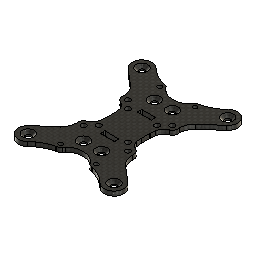
T_v2_Bottom_Plate_7_Inch_3mm (Autodesk Fusion 360 design; units mm, degrees)
Autodesk Fusion 360 part; units mm, degrees
sketch "Bottom Plate v2 3mm" plane through (0, 0, 0) normal (0, 0, 1) x (1, 0, 0)
  line L0 (23.8549, 2.6173) -> (23.8549, 4.2)
  arc A0 (38.0902, -44.8281) -> (37.3115, -43.7825) centre (33.725, -47.2663) ccw
  arc A1 (3.5774, -53.5563) -> (-5.1954, -43.2296) centre (-0.8133, -48.3966) cw
  arc A2 (24.6115, 1.8607) -> (23.8549, 2.6173) centre (24.2332, 2.239) cw
  line L1 (32.7104, -23.5665) -> (24.6115, -23.5665)
  arc A3 (16.0943, -15.706) -> (16.4474, -12.2676) centre (-17.5938, -10.5095) ccw
  arc A4 (40.5915, -46.4096) -> (38.0902, -44.8281) centre (40.7966, -43.3163) cw
  circle A5 centre (34.8621, 15.0393) radius 1.95
  arc A6 (23.8549, 4.2) -> (24.6115, 4.9567) centre (24.2332, 4.5783) cw
  arc A7 (41.2277, -2.9039) -> (40.8746, -6.3422) centre (74.9158, -8.1003) ccw
  line L2 (24.6115, -20.4705) -> (32.7104, -20.4705)
  arc A8 (47.7927, -25.5206) -> (51.1194, -33.5105) centre (59.6599, -25.267) ccw
  arc A9 (20.0105, 25.1727) -> (37.3115, 25.1727) centre (28.661, 33.5756) ccw
  arc A10 (24.6115, -23.5665) -> (23.8549, -22.8099) centre (24.2332, -23.1882) cw
  circle A11 centre (18.661, 0.6951) radius 1.75
  arc A12 (40.8746, -12.2676) -> (41.2277, -15.706) centre (74.9158, -10.5095) ccw
  line L3 (24.6115, 4.9567) -> (32.7104, 4.9567)
  arc A13 (33.467, 2.6173) -> (32.7104, 1.8607) centre (33.0887, 2.239) cw
  arc A14 (40.8746, -6.3422) -> (40.8775, -6.4049) centre (74.188, -4.8447) ccw
  arc A15 (23.8549, -21.2271) -> (24.6115, -20.4705) centre (24.2332, -20.8488) cw
  arc A16 (16.1379, -46.4846) -> (6.6741, -50.9212) centre (21.6796, -70.6178) ccw
  arc A17 (6.2139, -33.5209) -> (9.5318, -25.5307) centre (-2.3021, -25.3006) ccw
  circle A18 centre (38.661, 0.6951) radius 1.75
  arc A19 (-5.2039, 24.6271) -> (3.5715, 34.9515) centre (-0.8144, 29.7877) cw
  arc A20 (37.3115, -43.7825) -> (20.0105, -43.7825) centre (28.661, -52.1854) ccw
  circle A21 centre (22.4599, -33.6491) radius 1.95
  arc A22 (33.467, -22.8099) -> (32.7104, -23.5665) centre (33.0887, -23.1882) cw
  arc A23 (16.4474, -6.3422) -> (16.0943, -2.9039) centre (-17.5938, -8.1003) ccw
  line L4 (33.467, 4.2) -> (33.467, 2.6173)
  circle A24 centre (22.4599, 15.0393) radius 1.95
  line L5 (23.8549, -22.8099) -> (23.8549, -21.2271)
  circle A25 centre (38.661, -19.3049) radius 1.75
  arc A26 (40.8775, -12.2049) -> (40.8746, -12.2676) centre (74.188, -13.7651) ccw
  circle A27 centre (-0.8133, -48.3966) radius 1.95
  arc A28 (11.677, 2.3405) -> (9.5318, 6.9209) centre (13.411, 5.9451) cw
  arc A29 (53.7651, 34.9349) -> (62.5417, 24.6115) centre (58.1639, 29.7821) cw
  circle A30 centre (18.661, -19.3049) radius 1.75
  line L6 (32.7104, 1.8607) -> (24.6115, 1.8607)
  arc A31 (37.3115, 25.1727) -> (38.0902, 26.2183) centre (33.725, 28.6565) ccw
  arc A32 (19.2318, 26.2183) -> (20.0105, 25.1727) centre (23.5969, 28.6565) ccw
  arc A33 (32.7104, 4.9567) -> (33.467, 4.2) centre (33.0887, 4.5783) cw
  arc A34 (16.7304, 27.7997) -> (19.2318, 26.2183) centre (16.5253, 24.7065) cw
  arc A35 (45.6449, -20.9503) -> (47.7927, -25.5206) centre (43.911, -24.5549) cw
  arc A36 (32.7104, -20.4705) -> (33.467, -21.2271) centre (33.0887, -20.8488) cw
  circle A37 centre (43.911, -24.5549) radius 1.75
  circle A38 centre (43.911, 5.9451) radius 1.75
  line L7 (62.5417, 24.6115) -> (51.1194, 14.9007)
  line L8 (53.7651, -53.5447) -> (50.661, -50.9058)
  arc A39 (47.7927, 6.9108) -> (45.6449, 2.3405) centre (43.911, 5.9451) cw
  line L9 (33.467, -21.2271) -> (33.467, -22.8099)
  circle A40 centre (13.411, 5.9451) radius 1.75
  line L10 (-5.1954, -43.2296) -> (6.2139, -33.5209)
  line L11 (6.2139, 14.9111) -> (-5.2039, 24.6271)
  circle A41 centre (16.5253, -43.3163) radius 1.45
  arc A42 (9.5318, -25.5307) -> (11.677, -20.9503) centre (13.411, -24.5549) cw
  line L12 (6.6741, -50.9212) -> (3.5774, -53.5563)
  circle A43 centre (58.1534, 29.7732) radius 1.95
  line L13 (6.6357, 32.344) -> (6.6741, 32.3114)
  line L14 (50.661, 32.296) -> (53.7651, 34.9349)
  arc A44 (41.1841, -46.4846) -> (40.5915, -46.4096) centre (40.2607, -51.3986) ccw
  arc A45 (40.5915, 27.7997) -> (41.1841, 27.8748) centre (40.2607, 32.7888) ccw
  arc A46 (16.1379, 27.8748) -> (16.7304, 27.7997) centre (17.0613, 32.7888) ccw
  circle A47 centre (40.7966, -43.3163) radius 1.45
  arc A48 (11.677, -20.9503) -> (16.0943, -15.706) centre (9.3857, -14.5378) ccw
  arc A49 (50.661, -50.9058) -> (41.1841, -46.4846) centre (35.4926, -71.0521) ccw
  circle A50 centre (34.8621, -33.6491) radius 1.95
  circle A51 centre (58.1534, -48.383) radius 1.95
  line L15 (16.4474, -12.2676) -> (16.4474, -6.3422)
  arc A52 (16.0943, -2.9039) -> (11.677, 2.3405) centre (9.3857, -4.072) ccw
  arc A53 (51.1194, 14.9007) -> (47.7927, 6.9108) centre (59.7146, 6.6344) ccw
  arc A54 (41.1841, 27.8748) -> (50.661, 32.296) centre (35.4926, 52.4423) ccw
  circle A55 centre (-0.8133, 29.7868) radius 1.95
  arc A56 (16.7304, -46.4096) -> (16.1379, -46.4846) centre (17.0613, -51.3986) ccw
  arc A57 (38.0902, 26.2183) -> (40.5915, 27.7997) centre (40.7966, 24.7065) cw
  arc A58 (6.6741, 32.3114) -> (16.1379, 27.8748) centre (21.6796, 52.0079) ccw
  arc A59 (41.2277, -15.706) -> (45.6449, -20.9503) centre (47.9363, -14.5378) ccw
  arc A60 (45.6449, 2.3405) -> (41.2277, -2.9039) centre (47.9363, -4.072) ccw
  line L16 (51.1194, -33.5105) -> (62.5417, -43.2213)
  line L17 (3.5715, 34.9515) -> (6.6357, 32.344)
  circle A61 centre (13.411, -24.5549) radius 1.75
  arc A62 (20.0105, -43.7825) -> (19.2318, -44.8281) centre (23.5969, -47.2663) ccw
  circle A63 centre (40.7966, 24.7065) radius 1.45
  circle A64 centre (-9.1434, 59.8386) radius 1.95
  circle A65 centre (16.5253, 24.7065) radius 1.45
  arc A66 (9.5318, 6.9209) -> (6.2139, 14.9111) centre (-2.3625, 6.6657) ccw
  line L18 (40.8775, -6.4049) -> (40.8775, -12.2049)
  arc A67 (62.5417, -43.2213) -> (53.7651, -53.5447) centre (58.1664, -48.3941) cw
  arc A68 (19.2318, -44.8281) -> (16.7304, -46.4096) centre (16.5253, -43.3163) cw
extrude "Extrude1" add sketch "Bottom Plate v2 3mm" against normal blind 3 contours A0 A1 A3 A4 A7 A8 A9 A12 A14 A16 A17 A19 A20 A23 A26 A28 A29 A31 A32 A34 A35 L7 L8 A39 L10 L11 A42 L12 L13 L14 A44 A45 A46 A48 A49 L15 A52 A53 A54 A56 A57 A58 A59 A60 L16 L17 A62 A66 L18 A67 A68
hole "Hole1" at (-0.8133, 29.7868, 0) direction (0, 0, -1) diameter 4 depth 26 tip angle 118 countersink diameter 8 countersink angle 90
hole "Hole2" at (22.4599, 15.0393, 0) direction (0, 0, -1) diameter 4 depth 26 tip angle 118 countersink diameter 8 countersink angle 90
hole "Hole3" at (34.8621, 15.0393, 0) direction (0, 0, -1) diameter 4 depth 26 tip angle 118 countersink diameter 8 countersink angle 90
hole "Hole4" at (58.1534, 29.7732, 0) direction (0, 0, -1) diameter 4 depth 26 tip angle 118 countersink diameter 8 countersink angle 90
hole "Hole5" at (22.4599, -33.6491, 0) direction (0, 0, -1) diameter 4 depth 26 tip angle 118 countersink diameter 8 countersink angle 90
hole "Hole6" at (34.8621, -33.6491, 0) direction (0, 0, -1) diameter 4 depth 26 tip angle 118 countersink diameter 8 countersink angle 90
hole "Hole7" at (-0.8133, -48.3966, 0) direction (0, 0, -1) diameter 4 depth 26 tip angle 118 countersink diameter 8 countersink angle 90
hole "Hole8" at (58.1534, -48.383, 0) direction (0, 0, -1) diameter 4 depth 26 tip angle 118 countersink diameter 8 countersink angle 90
named bodies: "Bottom Plate 3mm"
